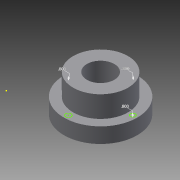
# Autodesk Inventor part: 7.2 Part #
Saved by Autodesk Inventor 2015 (Build 190159000, 159)
## iProperties
Created: 2015-03-16
Part Number: 7.2 Part #
Material: Generic
Document SubType Name: Modeling
Designer: PLTW-Stu-02
Density: 1 g/cm^3
Appearance: Default
Author: PLTW-Stu-02
Autodesk Inventor part; units mm, degrees
ref_plane "YZ Plane" through (0, 0, 0) normal (1, 0, 0) x (0, 1, 0)
ref_plane "XZ Plane" through (0, 0, 0) normal (0, 1, 0) x (-1, 0, 0)
ref_plane "XY Plane" through (0, 0, 0) normal (0, 0, 1) x (1, 0, 0)
sketch "Sketch1" plane through (0, 0, 0) normal (0, 1, 0) x (-1, 0, 0)
  circle A0 centre (-218.3045, -174.8397) radius 152.4
  circle A1 centre (-218.3045, -174.8397) radius 114.3
  circle A2 centre (-218.3045, -174.8397) radius 57.15
  point P0 (0, 0)
  dimension "d0" = 304.8
  dimension "d1" = 228.6
  dimension "d6" = 114.3
  constraints: 3 centre point, 2 coincident
  measures "d0" diameter of A0
  measures "d1" diameter of A1
  measures "d6" diameter of A2
extrude "Extrusion1" add sketch "Sketch1" along normal blind 63.5 contours A0
extrude "Extrusion2" add sketch "Sketch1" along normal blind 152.4 contours A1 | A2
sketch "Sketch2" plane through (218.3045, 152.4, -174.8397) normal (0, 1, 0) x (1, 0, 0)
  circle A0 centre (0, 0) radius 57.15
  point P0 (-218.3045, -174.8397)
  dimension "d7" = 114.3
  constraints: 1 centre point
  measures "d7" diameter of A0
extrude "Extrusion3" cut sketch "Sketch2" against normal through all
sketch "Sketch3" plane through (218.3045, 63.5, -174.8397) normal (0, 1, 0) x (1, 0, 0)
  circle A0 centre (133.5524, 0) radius 10.16
  circle A1 centre (0, 135.3792) radius 10.16
  circle A2 centre (-132.8036, 0) radius 10.16
  circle A3 centre (0, -134.7909) radius 11.3617
  point P0 (-218.3045, -174.8397)
  dimension "d10" = 20.32
  dimension "d11" = 20.32
  dimension "d12" = 20.32
  constraints: 4 centre point
  measures "d10" diameter of A0
  measures "d11" diameter of A1
  measures "d12" diameter of A2
body "Solid1"
